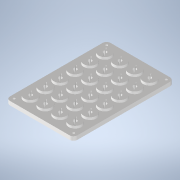
# Autodesk Inventor part: Omniscope_Base_v0
Saved by Autodesk Inventor 2022 (Build 260153000, 153)
## iProperties
Created: 2022-05-25
Part Number: Omniscope_Base_v0
Material: Generisch
Document SubType Name: Modeling
Designer: diederichbenedict
Density: 1 g/cm^3
Appearance: Vorgabe
Author: diederichbenedict
Autodesk Inventor part; units mm, degrees
ref_plane "YZ Plane" through (0, 0, 0) normal (1, 0, 0) x (0, 1, 0)
ref_plane "XZ Plane" through (0, 0, 0) normal (0, 1, 0) x (-1, 0, 0)
ref_plane "XY Plane" through (0, 0, 0) normal (0, 0, 1) x (1, 0, 0)
sketch "Skizze1" plane through (0, 0, 0) normal (0, 1, 0) x (-1, 0, 0)
  line L0 (-42.75, -63.75) -> (42.75, -63.75)
  line L1 (42.75, -63.75) -> (42.75, 63.75)
  line L2 (42.75, 63.75) -> (-42.75, 63.75)
  line L3 (-42.75, 63.75) -> (-42.75, -63.75)
  line L4 (-42.75, -63.75) -> (42.75, 63.75) construction
  line L5 (42.75, -63.75) -> (-42.75, 63.75) construction
  point P0 (0, 0)
  dimension "d0" = 85.5
  dimension "d1" = 127.5
  constraints: 12 end point, 2 midpoint, 2 parallel, 1 horizontal, 1 perpendicular
  measures "d0" distance of L2.end L1.end
  measures "d1" distance of L1.end L0.end
extrude "Extrusion1" add sketch "Skizze1" along normal blind 5
sketch "Skizze2" plane through (0, 5, 0) normal (0, 1, 0) x (1, 0, 0)
  line L0 (-42.75, 63.75) -> (-42.75, -63.75) projected
  line L1 (-42.75, -63.75) -> (42.75, -63.75) projected
  line L2 (42.75, -63.75) -> (42.75, 63.75) projected
  line L3 (42.75, 63.75) -> (-42.75, 63.75) projected
  circle A0 centre (-28.35, -47.25) radius 8
  line L4 (-21.85, -47.675) -> (-34.85, -47.675)
  line L5 (-34.85, -47.675) -> (-34.85, -46.825)
  line L6 (-34.85, -46.825) -> (-21.85, -46.825)
  line L7 (-21.85, -46.825) -> (-21.85, -47.675)
  line L8 (-21.85, -47.675) -> (-34.85, -46.825) construction
  line L9 (-34.85, -47.675) -> (-21.85, -46.825) construction
  point P0 (0, 0)
  dimension "d4" = 16
  dimension "d5" = 16.5
  dimension "d6" = 14.4
  dimension "d15" = 0.85
  dimension "d16" = 13
  constraints: 12 end point, 2 midpoint, 2 parallel, 1 centre point, 1 horizontal, 1 perpendicular
  measures "d4" diameter of A0
  measures "d5" distance from line of A0.centre L1
  measures "d6" distance from line of A0.centre L0
  measures "d15" distance between parallel lines of L6 L4
  measures "d16" horizontal distance of L6.end L4.end
extrude "Extrusion2" add sketch "Skizze2" along normal blind 3 contours A0 | L4 L5 L6 L7
fillet "Rundung1" radius 5 4 edges at (-42.75, 2.5, 63.75) (42.75, 2.5, 63.75) (42.75, 2.5, -63.75) (-42.75, 2.5, -63.75)
sketch "Skizze3" plane through (0, 8, 0) normal (0, 1, 0) x (1, 0, 0)
  circle A0 centre (-28.35, -47.25) radius 8 projected
  circle A1 centre (-28.35, -47.25) radius 8 projected
  arc A2 (-37.75, 63.75) -> (-42.75, 58.75) centre (-37.75, 58.75) ccw projected
  line L0 (-42.75, 58.75) -> (-42.75, -58.75) projected
  arc A3 (-42.75, -58.75) -> (-37.75, -63.75) centre (-37.75, -58.75) ccw projected
  line L1 (-37.75, -63.75) -> (37.75, -63.75) projected
  arc A4 (37.75, -63.75) -> (42.75, -58.75) centre (37.75, -58.75) ccw projected
  line L2 (42.75, -58.75) -> (42.75, 58.75) projected
  arc A5 (42.75, 58.75) -> (37.75, 63.75) centre (37.75, 58.75) ccw projected
  line L3 (37.75, 63.75) -> (-37.75, 63.75) projected
  point P0 (0, 0)
hole "Bohrung1" at (-28.35, 8, 47.25) direction (0, -1, 0) diameter 4.6 end through all
sketch "Skizze4" plane through (-28.35, 8, 47.25) normal (0, 1, 0) x (1, 0, 0)
  circle A0 centre (0, 0) radius 2.3 projected
  circle A1 centre (0, 0) radius 8 projected
  line L0 (6.6, -0.425) -> (-6.6, -0.425)
  line L1 (-6.6, -0.425) -> (-6.6, 0.425)
  line L2 (-6.6, 0.425) -> (6.6, 0.425)
  line L3 (6.6, 0.425) -> (6.6, -0.425)
  arc A2 (2.3, 0) -> (2.3, 0) centre (0, 0) ccw projected
  line L4 (6.6, -0.425) -> (-6.6, 0.425) construction
  line L5 (-6.6, -0.425) -> (6.6, 0.425) construction
  line L6 (3.4375, -5.6502) -> (-4.1337, 5.1626)
  line L7 (-4.1337, 5.1626) -> (-3.4375, 5.6502)
  line L8 (-3.4375, 5.6502) -> (4.1337, -5.1626)
  line L9 (4.1337, -5.1626) -> (3.4375, -5.6502)
  line L10 (3.4375, -5.6502) -> (-3.4375, 5.6502) construction
  line L11 (-4.1337, 5.1626) -> (4.1337, -5.1626) construction
  line L12 (3.4375, -5.6502) -> (16.6375, -5.6502) construction
  point P0 (28.35, 47.25)
  point P1 (-0.2212, -0.425)
  point P2 (0.8164, -0.425)
  point P3 (2.2604, -0.425)
  point P4 (2.2604, 0.425)
  point P5 (0.2212, 0.425)
  point P6 (-0.8164, 0.425)
  point P7 (-2.2604, 0.425)
  point P8 (-2.2604, -0.425)
  dimension "d25" = 13.2
  dimension "d26" = 0.85
  dimension "d35" = 13.2
  dimension "d36" = 125
  dimension "d37" = 0.85
  constraints: 26 end point, 4 midpoint, 4 parallel, 2 horizontal, 2 perpendicular, 1 equal length
  measures "d25" distance of L1.end L2.end
  measures "d26" distance of L0.end L1.end
  measures "d35" distance of L6.start L6.end
  measures "d36" angle of L12 L6
  measures "d37" distance of L6.end L7.end
extrude "Extrusion3" cut sketch "Skizze4" against normal blind 6 contours A0 L0 L8 L2 | L8 L2 L6 A0 | A0 L6 L7 L8 | L8 L0 L6 L2 | L8 L9 L6 A0 | A0 L6 L0 L8 | L6 L0 A0 L2
pattern_linear "Rechteckige Anordnung2" count 6 spacing 18.9 along (0, 0, -1) count 4 spacing 18.9 along (1, 0, 0) of "Bohrung1", "Extrusion3", "Extrusion2"
sketch "Skizze5" plane through (0, 0, 0) normal (0, -1, 0) x (1, 0, 0)
  circle A0 centre (28.35, -47.25) radius 2.3 projected
  circle A1 centre (28.35, -28.35) radius 2.3 projected
  circle A2 centre (28.35, -9.45) radius 2.3 projected
  circle A3 centre (28.35, 9.45) radius 2.3 projected
  circle A4 centre (28.35, 28.35) radius 2.3 projected
  circle A5 centre (28.35, 47.25) radius 2.3 projected
  circle A6 centre (9.45, -47.25) radius 2.3 projected
  circle A7 centre (9.45, -28.35) radius 2.3 projected
  circle A8 centre (9.45, -9.45) radius 2.3 projected
  circle A9 centre (9.45, 9.45) radius 2.3 projected
  circle A10 centre (9.45, 28.35) radius 2.3 projected
  circle A11 centre (9.45, 47.25) radius 2.3 projected
  circle A12 centre (-9.45, -47.25) radius 2.3 projected
  circle A13 centre (-9.45, -28.35) radius 2.3 projected
  circle A14 centre (-9.45, -9.45) radius 2.3 projected
  circle A15 centre (-9.45, 9.45) radius 2.3 projected
  circle A16 centre (-9.45, 28.35) radius 2.3 projected
  circle A17 centre (-9.45, 47.25) radius 2.3 projected
  circle A18 centre (-28.35, -47.25) radius 2.3 projected
  circle A19 centre (-28.35, -28.35) radius 2.3 projected
  circle A20 centre (-28.35, -9.45) radius 2.3 projected
  circle A21 centre (-28.35, 9.45) radius 2.3 projected
  circle A22 centre (-28.35, 28.35) radius 2.3 projected
  circle A23 centre (-28.35, 47.25) radius 2.3 projected
  arc A24 (-42.75, -58.75) -> (-37.75, -63.75) centre (-37.75, -58.75) ccw projected
  line L0 (37.75, -63.75) -> (-37.75, -63.75) projected
  arc A25 (37.75, -63.75) -> (42.75, -58.75) centre (37.75, -58.75) ccw projected
  line L1 (42.75, 58.75) -> (42.75, -58.75) projected
  arc A26 (42.75, 58.75) -> (37.75, 63.75) centre (37.75, 58.75) ccw projected
  line L2 (-37.75, 63.75) -> (37.75, 63.75) projected
  arc A27 (-37.75, 63.75) -> (-42.75, 58.75) centre (-37.75, 58.75) ccw projected
  line L3 (-42.75, -58.75) -> (-42.75, 58.75) projected
  circle A28 centre (28.35, 47.25) radius 2.3 projected
  arc A29 (29.2984, -45.1546) -> (26.7054, -48.8578) centre (28.35, -47.25) ccw projected
  line L4 (30.65, 47.25) -> (26.05, 47.25)
  line L5 (26.05, 47.25) -> (26.05, -47.25)
  line L6 (26.05, -47.25) -> (30.65, -47.25)
  line L7 (30.65, -47.25) -> (30.65, 47.25)
  circle A30 centre (9.45, 47.25) radius 2.3 projected
  line L8 (11.75, 47.25) -> (7.15, 47.25)
  line L9 (7.15, 47.25) -> (7.15, -47.25)
  line L10 (7.15, -47.25) -> (11.75, -47.25)
  line L11 (11.75, -47.25) -> (11.75, 47.25)
  circle A31 centre (-9.45, 47.25) radius 2.3 projected
  line L12 (-7.15, 47.25) -> (-11.75, 47.25)
  line L13 (-11.75, 47.25) -> (-11.75, -47.25)
  line L14 (-11.75, -47.25) -> (-7.15, -47.25)
  line L15 (-7.15, -47.25) -> (-7.15, 47.25)
  arc A32 (-29.2984, 45.1546) -> (-26.7054, 48.8578) centre (-28.35, 47.25) ccw projected
  line L16 (-26.05, 47.25) -> (-30.65, 47.25)
  line L17 (-30.65, 47.25) -> (-30.65, -47.25)
  line L18 (-30.65, -47.25) -> (-26.05, -47.25)
  line L19 (-26.05, -47.25) -> (-26.05, 47.25)
  line L20 (-42.75, -58.75) -> (-42.75, 58.75) projected
  line L21 (28.35, -44.95) -> (-42.75, -44.95)
  line L22 (-42.75, -44.95) -> (-42.75, -49.55)
  line L23 (-42.75, -49.55) -> (28.35, -49.55)
  line L24 (28.35, -49.55) -> (28.35, -44.95)
  point P0 (0, 0)
  point P1 (26.05, -44.95)
  point P2 (11.75, -44.95)
  point P3 (7.15, -44.95)
  point P4 (-7.15, -44.95)
  point P5 (-11.75, -44.95)
  point P6 (-26.05, -44.95)
  point P7 (-30.65, -44.95)
  constraints: 40 end point, 10 parallel, 7 point on line, 6 horizontal alignment, 5 horizontal, 5 perpendicular, 3 point on circle, 6 other
extrude "Extrusion4" cut sketch "Skizze5" against normal blind 2 contours L6 L24 A0 | A0 L24 L6 | A0 L21 L5 A1 L7 | L23 A6 L11 L21 L5 A0 | A0 L6 L24 | L6 A0 L24 | A1 | A1 L5 A2 L7 | A0 L5 L21 | L23 A12 L15 L21 L9 A6 | A6 L10 | A2 | A2 L5 A3 L7 | L9 L21 A6 | A6 L10 | A6 L21 L11 | L23 A18 L19 L21 L13 A12 | A12 L14 | A3 | A3 L5 A4 L7 | L21 L9 A7 L11 | L13 L21 A12 | A12 L14 | A12 L21 L15 | L23 L3 L21 L17 A18 | A18 L18 | A4 | A4 L5 A5 L7 | A7 | A7 L9 A8 L11 | L21 L13 A13 L15 | L17 L21 A18 | A18 L18 | A18 L21 L19 | A5 L4 | A8 | A8 L9 A9 L11 | A13 | A13 L13 A14 L15 | L21 L17 A19 L19 | A9 | A9 L9 A10 L11 | A14 | A14 L13 A15 L15 | A19 | A19 L17 A20 L19 | A10 | A10 L9 A11 L11 | A15 | A15 L13 A16 L15 | A20 | A20 L17 A21 L19 | A11 L8 | A16 | A16 L13 A17 L15 | A21 | A21 L17 A22 L19 | A17 L12 | A22 | A22 L17 A23 L19 | A23 L16 picked at (27.6056, 47.0665) picked at (8.7056, 47.0665) picked at (-10.1944, 47.0665) picked at (-28.6661, 46.5515)
sketch "Skizze6" plane through (0, 5, 0) normal (0, 1, 0) x (1, 0, 0)
  circle A0 centre (28.35, 47.25) radius 8 projected
  circle A1 centre (28.35, 28.35) radius 8 projected
  circle A2 centre (28.35, 9.45) radius 8 projected
  circle A3 centre (28.35, -9.45) radius 8 projected
  circle A4 centre (28.35, -28.35) radius 8 projected
  circle A5 centre (28.35, -47.25) radius 8 projected
  circle A6 centre (9.45, 47.25) radius 8 projected
  circle A7 centre (9.45, 28.35) radius 8 projected
  circle A8 centre (9.45, 9.45) radius 8 projected
  circle A9 centre (9.45, -9.45) radius 8 projected
  circle A10 centre (9.45, -28.35) radius 8 projected
  circle A11 centre (9.45, -47.25) radius 8 projected
  circle A12 centre (-9.45, 47.25) radius 8 projected
  circle A13 centre (-9.45, 28.35) radius 8 projected
  circle A14 centre (-9.45, 9.45) radius 8 projected
  circle A15 centre (-9.45, -9.45) radius 8 projected
  circle A16 centre (-9.45, -28.35) radius 8 projected
  circle A17 centre (-9.45, -47.25) radius 8 projected
  circle A18 centre (-28.35, 47.25) radius 8 projected
  circle A19 centre (-28.35, 28.35) radius 8 projected
  circle A20 centre (-28.35, 9.45) radius 8 projected
  circle A21 centre (-28.35, -9.45) radius 8 projected
  circle A22 centre (-28.35, -28.35) radius 8 projected
  arc A23 (-37.75, 63.75) -> (-42.75, 58.75) centre (-37.75, 58.75) ccw projected
  line L0 (-42.75, 58.75) -> (-42.75, -58.75) projected
  arc A24 (-42.75, -58.75) -> (-37.75, -63.75) centre (-37.75, -58.75) ccw projected
  line L1 (-37.75, -63.75) -> (37.75, -63.75) projected
  arc A25 (37.75, -63.75) -> (42.75, -58.75) centre (37.75, -58.75) ccw projected
  line L2 (42.75, -58.75) -> (42.75, 58.75) projected
  arc A26 (42.75, 58.75) -> (37.75, 63.75) centre (37.75, 58.75) ccw projected
  line L3 (37.75, 63.75) -> (-37.75, 63.75) projected
  circle A27 centre (-28.35, -47.25) radius 8 projected
  point P0 (0, 0)
hole "Bohrung2" at (-37.75, 5, 58.75) at (37.75, 5, 58.75) at (-37.75, 5, -58.75) at (37.75, 5, -58.75) direction (0, -1, 0) diameter 2.8 end through all
